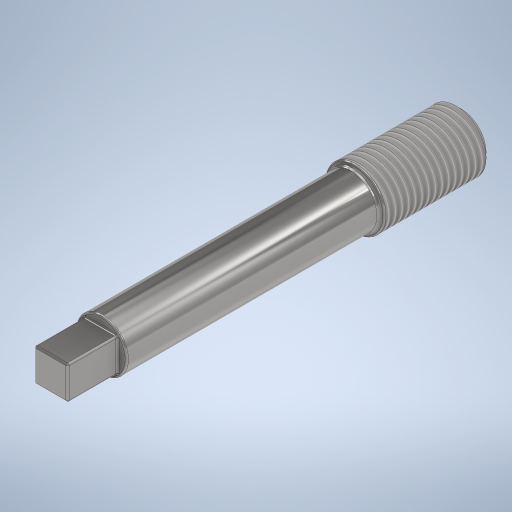
# Autodesk Inventor part: shaft
Saved by Autodesk Inventor 2024 (Build 280153000, 153)
## iProperties
Created: 2024-03-24
Part Number: shaft
Material: Generic
Document SubType Name: Sheet Metal
Designer: MSI-C
Density: 1 g/cm^3
Sheet Metal Rule: Default_mm
Appearance: Steel - Polished
Mass: 23.6782 g
Surface Area: 66.1957 cm^2
Volume: 23.6782 cm^3
Author: MSI-C
Autodesk Inventor part; units mm, degrees
ref_plane "YZ Plane" through (0, 0, 0) normal (1, 0, 0) x (0, 1, 0)
ref_plane "XZ Plane" through (0, 0, 0) normal (0, 1, 0) x (-1, 0, 0)
ref_plane "XY Plane" through (0, 0, 0) normal (0, 0, 1) x (1, 0, 0)
sketch "Sketch1" plane through (0, 0, 0) normal (0, 0, 1) x (1, 0, 0)
  circle A0 centre (0, 0) radius 7.75
  circle A1 centre (0, 0) radius 9
  dimension "d0" = 15.5
  dimension "d34" = 18
  constraints: 2 centre point, 2 coincident
  measures "d0" diameter of A0
  measures "d34" diameter of A1
extrude "Extrusion1" add sketch "Sketch1" along normal blind 108 contours A0
sketch "Sketch2" plane through (0, 0, 108) normal (0, 0, 1) x (1, 0, 0)
  line L0 (5, 5) -> (-5, 5)
  line L1 (-5, 5) -> (-5, -5)
  line L2 (-5, -5) -> (5, -5)
  line L3 (5, -5) -> (5, 5)
  line L4 (5, 5) -> (-5, -5) construction
  line L5 (-5, 5) -> (5, -5) construction
  point P0 (0, 0)
  dimension "d3" = 10
  dimension "d4" = 10
  constraints: 12 end point, 2 midpoint, 2 parallel, 1 horizontal, 1 perpendicular
  measures "d3" distance of L0.start L0.end
  measures "d4" distance of L2.end L0.start
extrude "Extrusion2" add sketch "Sketch2" along normal blind 15
sketch "Sketch3" plane through (0, 0, 0) normal (0, 0, -1) x (-1, 0, 0)
  line L0 (3.5, -3.5) -> (-3.5, -3.5)
  line L1 (-3.5, -3.5) -> (-3.5, 3.5)
  line L2 (-3.5, 3.5) -> (3.5, 3.5)
  line L3 (3.5, 3.5) -> (3.5, -3.5)
  line L4 (3.5, -3.5) -> (-3.5, 3.5) construction
  line L5 (-3.5, -3.5) -> (3.5, 3.5) construction
  point P0 (0, 0)
  dimension "d13" = 7
  dimension "d14" = 7
  constraints: 12 end point, 2 midpoint, 2 parallel, 1 horizontal, 1 perpendicular
  measures "d13" distance of L0.start L0.end
  measures "d14" distance of L0.end L1.end
extrude "Extrusion3" cut sketch "Sketch3" against normal blind 5
extrude "Extrusion5" add sketch "Sketch1" along normal blind 32
fillet "Face Fillet1" radius 1 1 edges at (-7.75, 0, 32)
fillet "Fillet7" radius 0.5 10 edges at (-9, 0, 32) (-7.75, 0, 108) (5, -5, 115.5) (-5, -5, 115.5) (5, 5, 115.5) (-5, 5, 115.5) (3.5, 0, 0) (0, -3.5, 0) (-3.5, 0, 0) (0, 3.5, 0)
chamfer "Chamfer5" distance 0.5 angle 45 8 edges at (-5, 0, 123) (-4.8536, -4.8536, 123) (0, -5, 123) (4.8536, -4.8536, 123) (5, 0, 123) (4.8536, 4.8536, 123) (0, 5, 123) (-4.8536, 4.8536, 123)
fillet "Fillet9" radius 0.5 8 edges at (-4.8536, -4.8536, 108) (-5, 0, 108) (-4.8536, 4.8536, 108) (0, 5, 108) (4.8536, 4.8536, 108) (5, 0, 108) (4.8536, -4.8536, 108) (0, -5, 108)
fillet "Fillet10" radius 0.5 4 edges at (0, 3.5, 5) (0, -3.5, 5) (3.5, 0, 5) (-3.5, 0, 5)
thread "Thread5" size "TR18x2" class "7e" standard "ISO Metric Trapezoidal Threads" length 32
chamfer "Chamfer6" distance 1.5 angle 45 1 edges at (-9, 0, 0)
sketch "Sketch5" plane through (0, 0, 0) normal (0, 1, 0) x (-1, 0, 0)
  point P0 (0, 0)
sketch "Sketch6" plane through (0, 0, 0) normal (0, 1, 0) x (-1, 0, 0)
  point P0 (0, 0)
equation "\"BendRadius\" = Thickness"
equation "\"BendReliefWidth\" = Thickness"
equation "\"BendReliefDepth\" = 0.5 * Thickness"
equation "\"CornerReliefSize\" = 4 * Thickness"
equation "\"MinimumRemnant\" = 2 * Thickness"
equation "\"TransitionRadius\" = BendRadius"
equation "\"JacobiRadiusSize\" = BendRadius"
equation "\"GapSize\" = Thickness"
equation "\"Thickness\" = 0.5"
body "Solid1"
